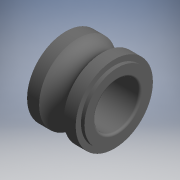
# Autodesk Inventor part: F624ZZ Inner Ring
Saved by Autodesk Inventor 2017.3 (Build 213256000, 256)
## iProperties
Part Number: F624ZZ Inner Ring
Material: Generic
Catalog Web Link: www.cadenas.de
Description: shielded_type_zz_zzs_IR-
Vendor: NSK_RB
Document SubType Name: Modeling
Designer: partserver
Manufacturer: NSK_RB
Mass: 0.102438 g
Surface Area: 2.209 cm^2
Volume: 0.102438 cm^3
Density: 1 g/cm^3
Appearance: PSOLRGB-128-128-128
Category: PARTsolutions
Company: NSK_RB
Title: F624ZZ Inner Ring
Author: Cadenas PARTsolutions
PSOL_IDENT_0: {$CADENAS_DATA\23d-libs\nsk_rb\roller_bearings\deep_groove_bb\exstra_small_miniatur_bb\metric_design
PSOL_IDENT_1: _with_flange\shielded_type_zz_zzs_ir_1.prj},192 {VTYP=3D},{NB=F624ZZ Inner Ring},{LINA=F624ZZ Inner
PSOL_IDENT_2: Ring},{NN=shielded_type_zz_zzs_IR},{DATE=16.07.2021 00:25:32},{GEOMDATE=04.01.2008 00:00:00},{VERSIO
PSOL_IDENT_3: N=},{LINEID=230},{WBVAR=},{WBNUMERIC=}  {NB=F624ZZ Inner Ring},{LINA=F624ZZ Inner Ring},{KT=DUMMY},{
PSOL_IDENT_4: IDNR=},{STAN=},{ORDER=F624ZZ},{SD=4.0},{X=4.0},{D=13},{DD=13},{DD1=0.0},{D2=15.0},{DD2=15.0},{B=0.0}
PSOL_IDENT_5: ,{B1=5.0},{CC1=0.0},{C2=1.0},{CC2=1.0},{R=0.00},{R1=0.20},{DI1=6.95},{DI2=6.00},{SDE1=10.45},{SDE2=1
PSOL_IDENT_6: 1.30},{CR1=1300},{COR1=485},{CR2=133},{COR2=49.0},{LG=40000},{LO=48000},{DA=0.0},{DB=6.0},{RA=0.00},
PSOL_IDENT_7: {RB=0.20},{MASS=3.53},{SC=1},{N=7}
NB: F624ZZ Inner Ring
NN: shielded_type_zz_zzs_IR
NBSYN: $ORDER. Inner Ring
LINA: F624ZZ Inner Ring
CATALOG: NSK Rolling Bearing
ORDER: F624ZZ
SD: 4
X: 4
D: 13
DD: 13
DD1: 0
D2: 15
DD2: 15
B: 0
B1: 5
CC1: 0
C2: 1
CC2: 1
R: 0
R1: 0.2
DI1: 6.95
DI2: 6
SDE1: 10.45
SDE2: 11.3
CR1: 1300
COR1: 485
CR2: 133
COR2: 49
LG: 40000
LO: 48000
DA: 0
DB: 6
RA: 0
RB: 0.2
MASS: 3.53
SC: 1
SUPPLIER: NSK_RB
ARTICLENO: F624ZZ Inner Ring
BOMINFO: F624ZZ Inner Ring
CREATOR: CADENAS GmbH
Autodesk Inventor part; units mm, degrees
sketch "Sketch_2" plane through (0, 0, 0) normal (0, 0, 1) x (1, 0, 0)
  line L0 (5, 0) -> (0, 0)
  arc A0 (0, 2.2) -> (0.2, 2) centre (0.2, 2.2) ccw
  line L1 (0.2, 2) -> (4.8, 2)
  arc A1 (4.8, 2) -> (5, 2.2) centre (4.8, 2.2) ccw
  line L2 (5, 2.2) -> (5, 3)
  line L3 (5, 3) -> (4.6875, 3)
  line L4 (4.6875, 3) -> (4.6875, 3.475)
  line L5 (4.6875, 3.475) -> (3.6054, 3.475)
  arc A2 (1.3946, 3.475) -> (3.6054, 3.475) centre (2.5, 4.25) ccw
  line L6 (1.3946, 3.475) -> (0.3125, 3.475)
  line L7 (0.3125, 3.475) -> (0.3125, 3)
  line L8 (0.3125, 3) -> (0, 3)
  line L9 (0, 3) -> (0, 2.2)
  constraints: 20 end point, 6 point on circle, 3 centre point
revolve "Revolution1" add sketch "Sketch_2" angle 360 about axis through (5, 0, 0) along (1, 0, 0)
ref_plane "ip_st_1_1_XY" through (2.5, 4.25, 0) normal (1, 0, 0) x (0, 0, -1)
ref_plane "ip_st_1_1_YZ" through (2.5, 4.25, 0) normal (0, 0, -1) x (0, 1, 0)
ref_plane "ip_st_1_1_ZX" through (2.5, 4.25, 0) normal (0, 1, 0) x (1, 0, 0)
ref_plane "ip_st_1_2_XY" through (2.5, 2.6498, 3.3228) normal (1, 0, 0) x (0, 0, -1)
ref_plane "ip_st_1_2_YZ" through (2.5, 2.6498, 3.3228) normal (0, 0, -1) x (0, 1, 0)
ref_plane "ip_st_1_2_ZX" through (2.5, 2.6498, 3.3228) normal (0, 1, 0) x (1, 0, 0)
ref_plane "ip_st_1_3_XY" through (2.5, -0.9457, 4.1434) normal (1, 0, 0) x (0, 0, -1)
ref_plane "ip_st_1_3_YZ" through (2.5, -0.9457, 4.1434) normal (0, 0, -1) x (0, 1, 0)
ref_plane "ip_st_1_3_ZX" through (2.5, -0.9457, 4.1434) normal (0, 1, 0) x (1, 0, 0)
ref_plane "ip_st_1_4_XY" through (2.5, -3.8291, 1.844) normal (1, 0, 0) x (0, 0, -1)
ref_plane "ip_st_1_4_YZ" through (2.5, -3.8291, 1.844) normal (0, 0, -1) x (0, 1, 0)
ref_plane "ip_st_1_4_ZX" through (2.5, -3.8291, 1.844) normal (0, 1, 0) x (1, 0, 0)
ref_plane "ip_st_1_5_XY" through (2.5, -3.8291, -1.844) normal (1, 0, 0) x (0, 0, -1)
ref_plane "ip_st_1_5_YZ" through (2.5, -3.8291, -1.844) normal (0, 0, -1) x (0, 1, 0)
ref_plane "ip_st_1_5_ZX" through (2.5, -3.8291, -1.844) normal (0, 1, 0) x (1, 0, 0)
ref_plane "ip_st_1_6_XY" through (2.5, -0.9457, -4.1434) normal (1, 0, 0) x (0, 0, -1)
ref_plane "ip_st_1_6_YZ" through (2.5, -0.9457, -4.1434) normal (0, 0, -1) x (0, 1, 0)
ref_plane "ip_st_1_6_ZX" through (2.5, -0.9457, -4.1434) normal (0, 1, 0) x (1, 0, 0)
ref_plane "ip_st_1_7_XY" through (2.5, 2.6498, -3.3228) normal (1, 0, 0) x (0, 0, -1)
ref_plane "ip_st_1_7_YZ" through (2.5, 2.6498, -3.3228) normal (0, 0, -1) x (0, 1, 0)
ref_plane "ip_st_1_7_ZX" through (2.5, 2.6498, -3.3228) normal (0, 1, 0) x (1, 0, 0)
ref_plane "ip_st_1a_XY" through (0, 0, 0) normal (1, 0, 0) x (0, 0, -1)
ref_plane "ip_st_1a_YZ" through (0, 0, 0) normal (0, 0, -1) x (0, 1, 0)
ref_plane "ip_st_1a_ZX" through (0, 0, 0) normal (0, 1, 0) x (1, 0, 0)
ref_plane "ip_st_2a_XY" through (0.3125, 0, 0) normal (1, 0, 0) x (0, 0, -1)
ref_plane "ip_st_2a_YZ" through (0.3125, 0, 0) normal (0, 0, -1) x (0, 1, 0)
ref_plane "ip_st_2a_ZX" through (0.3125, 0, 0) normal (0, 1, 0) x (1, 0, 0)
body "Solid1"
